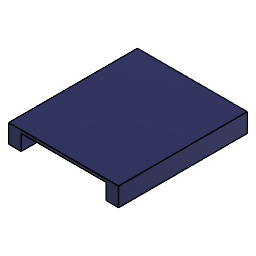
plytka (Autodesk Fusion 360 design; units mm, degrees)
part number: 2025-11-20-18-44-38-071
Autodesk Fusion 360 part; units mm, degrees
sketch "Szkic1" plane through (0, 0, 0) normal (0, 0, 1) x (1, 0, 0)
  line L0 (0, 0) -> (70, 0)
  line L1 (70, 0) -> (70, 82)
  line L2 (70, 82) -> (0, 82)
  line L3 (0, 82) -> (0, 0)
  dimension "d1" = 70
  dimension "d2" = 82
  constraint horizontal L0
  constraint vertical L1
  constraint horizontal L2
  constraint vertical L3
  constraint coincident L0.start L3.end
  measures "d1" distance of L0.start L0.end
  measures "d2" distance of L0.start L2.end
extrude "Wyciągnięcie proste1" add sketch "Szkic1" along normal blind 12
sketch "Szkic2" plane through (0, 0, 0) normal (0, 0, -1) x (1, 0, 0)
  line L0 (0, 0) -> (0, -82)
  line L1 (0, -82) -> (70, -82)
  line L2 (70, -82) -> (70, 0)
  line L3 (70, 0) -> (0, 0)
  line L4 (8, 0) -> (62, 0)
  line L5 (62, 0) -> (62, -82)
  line L6 (62, -82) -> (8, -82)
  line L7 (8, -82) -> (8, 0)
  dimension "d5" = 54
  dimension "d6" = 82
  constraint horizontal L4
  constraint vertical L5
  constraint horizontal L6
  constraint vertical L7
  constraint coincident L3 L4.start
  measures "d5" distance of L4.start L4.end
  measures "d6" distance of L4.start L6.end
extrude "Wyciągnięcie proste2" cut sketch "Szkic2" against normal blind 10 contours L1 L3 L4 L5 L6 L7
named bodies: "plytka"
